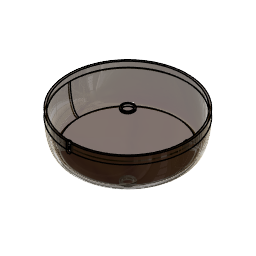
OuterSheelBase2_v7 (Autodesk Fusion 360 design; units mm, degrees)
Autodesk Fusion 360 part; units mm, degrees
sketch "Sketch1" plane through (0, 0, 0) normal (0, 0, 1) x (1, 0, 0)
  circle A0 centre (0, 0) radius 66
  circle A1 centre (0, 0) radius 64
  line L0 (35.2025, -35.2025) -> (-35.2025, -35.2025) construction
  line L1 (-35.2025, -35.2025) -> (-35.2025, 35.2025) construction
  line L2 (-35.2025, 35.2025) -> (35.2025, 35.2025) construction
  line L3 (35.2025, 35.2025) -> (35.2025, -35.2025) construction
  line L4 (35.2025, -35.2025) -> (-35.2025, 35.2025) construction
  line L5 (-35.2025, -35.2025) -> (35.2025, 35.2025) construction
  circle A2 centre (-35.2025, 35.2025) radius 5.1
  circle A3 centre (35.2025, 35.2025) radius 5.1
  circle A4 centre (-35.2025, -35.2025) radius 5.1
  circle A5 centre (35.2025, -35.2025) radius 5.1
  circle A6 centre (-35.2025, 35.2025) radius 6.6
  circle A7 centre (-35.2025, -35.2025) radius 6.6
  circle A8 centre (35.2025, -35.2025) radius 6.6
  circle A9 centre (35.2025, 35.2025) radius 6.6
  dimension "d1" = 132
  dimension "d2" = 2
  dimension "d7" = 70.405
  dimension "d8" = 70.405
  dimension "d9" = 10.2
  dimension "d10" = 10.2
  dimension "d11" = 10.2
  dimension "d12" = 10.2
  dimension "d15" = 1.5
  dimension "d17" = 360
  constraint coincident A0.centre A1.centre
  constraint horizontal L0
  constraint perpendicular L0 L1
  constraint parallel L0 L2
  constraint parallel L1 L3
  constraint coincident L4 A0.centre
  constraint coincident L5 A0.centre
  constraint coincident L1.end L2.start
  constraint coincident L2.end L3.start
  constraint coincident L0.end L1.start
  constraint coincident L0.start L3.end
  constraint concentric A2 A6
  measures "d1" diameter of A0
  measures "d2" distance of A0 A1
  measures "d7" distance of L1.end L2.end
  measures "d8" distance of L0.end L1.end
  measures "d9" diameter of A2
  measures "d10" diameter of A3
  measures "d11" diameter of A4
  measures "d12" diameter of A5
  measures "d15" distance of A2 A6
extrude "Extrude1" add sketch "Sketch1" against normal blind 2 contours A0 | A1 | A2 | A3 | A4 | A5 | A6 | A7 | A8 | A9
extrude "Extrude2" add sketch "Sketch1" along normal blind 30 contours A0
extrude "Extrude3" cut sketch "Sketch1" against normal blind 1 contours A2 | A3 | A4 | A5
extrude "Extrude4" add sketch "Sketch1" along normal blind 1.5 contours A6 | A7 | A8 | A9
sketch "Sketch2" plane through (0, 0, 0) normal (0, 1, 0) x (1, 0, 0)
  line L0 (0, 0) -> (0, -30) construction
  circle A0 centre (0, -27.5) radius 2.5
  line L1 (-2.5, -30) -> (2.5, -30)
  line L2 (2.5, -30) -> (2.5, -27.5)
  line L3 (-2.5, -30) -> (-2.5, -27.5)
  dimension "d20" = 5
  dimension "d21" = 5
  constraint coincident L0.start origin
  constraint vertical L0
  constraint coincident L0 A0.centre
  constraint midpoint L0.end L1
  constraint perpendicular L0 L1
  constraint coincident A0 L2.end
  constraint tangent A0 L2
  constraint coincident A0 L3.end
  constraint tangent A0 L3
  constraint tangent A0 L1
  measures "d20" diameter of A0
  measures "d21" distance of L1.start L1.end
extrude "Extrude5" cut sketch "Sketch2" against normal blind 110
extrude "Extrude6" add 1 faces at (-5.6911, -64.93, 30) along direction (0, 0, 1) blind 6
fillet "Fillet1" offset 10 second offset 30 1 edges at (-59.669, -23.1434, 0) measured on face at (-10.1215, -10.2378, 0)
fillet "Fillet2" offset 10 second offset 30 1 edges at (-61.5336, 23.8666, -2) measured on face at (19.2692, 15.933, -2)
equation "d1 = ( 66 * 2 ) * 1 mm"
